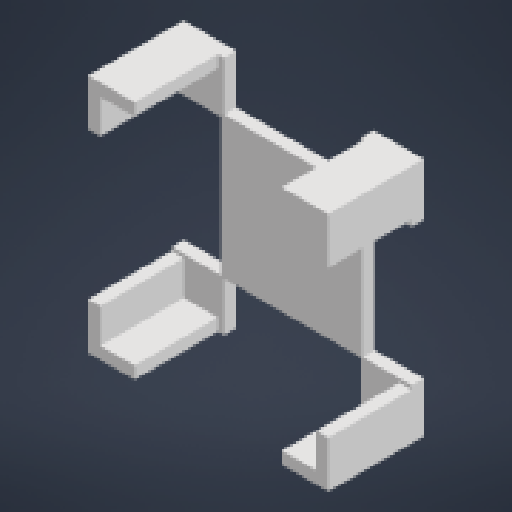
# Autodesk Inventor part: SistemaLiberacion2.2
Saved by Autodesk Inventor 2026.1 (Build 301233000, 233)
## iProperties
Created: 2025-11-13
Part Number: SistemaLiberacion2.2
Material: Genérico
Document SubType Name: Modeling
Designer: usuario
Density: 1 g/cm^3
Appearance: Valor por defecto
Author: usuario
Autodesk Inventor part; units mm, degrees
ref_plane "YZ Plane" through (0, 0, 0) normal (1, 0, 0) x (0, 1, 0)
ref_plane "XZ Plane" through (0, 0, 0) normal (0, 1, 0) x (-1, 0, 0)
ref_plane "XY Plane" through (0, 0, 0) normal (0, 0, 1) x (1, 0, 0)
sketch "Boceto1" plane through (0, 0, 0) normal (0, 0, 1) x (1, 0, 0)
  line L0 (-49, 49) -> (-49, -49)
  line L1 (-49, -49) -> (49, -49)
  line L2 (49, -49) -> (49, 49)
  line L3 (49, 49) -> (-49, 49)
  line L4 (-49, 49) -> (49, -49) construction
  line L5 (-49, -49) -> (49, 49) construction
  line L6 (-44, 44) -> (-44, -44)
  line L7 (-44, -44) -> (44, -44)
  line L8 (44, -44) -> (44, 44)
  line L9 (44, 44) -> (-44, 44)
  line L10 (-44, 44) -> (44, -44) construction
  line L11 (-44, -44) -> (44, 44) construction
  line L12 (-49, -30) -> (49, -30)
  line L13 (-49, 30) -> (49, 30)
  line L14 (-30, -49) -> (-30, 49)
  line L15 (30, -49) -> (30, 49)
  point P0 (0, 0)
  point P1 (0, -30)
  point P2 (0, -49)
  point P3 (-30, 44)
  point P4 (-44, 30)
  point P5 (30, 44)
  point P6 (44, 30)
  point P7 (30, -44)
  point P8 (44, -30)
  point P9 (-30, -44)
  point P10 (-44, -30)
  dimension "d0" = 98
  dimension "d1" = 98
  dimension "d2" = 5
  dimension "d3" = 5
  dimension "d8" = 19
  dimension "d10" = 19
  dimension "d11" = 19
  dimension "d18" = 19
  constraints: 32 end point, 8 point on line, 6 midpoint, 6 perpendicular, 4 parallel, 1 vertical
  measures "d0" distance of L0.start L0.end
  measures "d1" distance of L1.end L0.end
  measures "d2" distance between parallel lines of L1 L7
  measures "d3" distance between parallel lines of L8 L2
  measures "d8" distance of point (0, -30) point (0, -49)
  measures "d10" distance between parallel lines of L14 L0
  measures "d11" distance between parallel lines of L2 L15
  measures "d18" distance between parallel lines of L3 L13
extrude "Extrusión1" add sketch "Boceto1" against normal blind 34 contours L3 L14 L9 L6 L13 L0 | L12 L6 L7 L14 L1 L0 | L3 L2 L13 L8 L9 L15 | L15 L7 L8 L12 L2 L1
sketch "Boceto2" plane through (0, 0, -34) normal (0, 0, -1) x (-1, 0, 0)
  line L0 (49, 49) -> (-49, 49) projected
  line L1 (-49, -49) -> (49, -49) projected
  line L2 (-49, 49) -> (49, 49)
  line L3 (49, 49) -> (49, -49)
  line L4 (49, -49) -> (-49, -49)
  line L5 (-49, -49) -> (-49, 49)
  line L6 (49, -30) -> (44, -30) projected
  line L7 (49, 26) -> (49, -30)
  line L8 (-49, -30) -> (-49, 26)
  line L9 (30, 49) -> (-26, 49)
  line L10 (30, -49) -> (-30, -49)
  line L11 (-28.5, -49) -> (27.5, -49)
  line L12 (27.5, -49) -> (27.5, -34)
  line L13 (27.5, -34) -> (-28.5, -34)
  line L14 (-28.5, -34) -> (-28.5, -49)
  line L15 (-28.5, 34) -> (27.5, 34)
  line L16 (27.5, 34) -> (27.5, 49)
  line L17 (27.5, 49) -> (-28.5, 49)
  line L18 (-28.5, 49) -> (-28.5, 34)
  line L19 (-49, -28.5) -> (-34, -28.5)
  line L20 (-34, -28.5) -> (-34, 27.5)
  line L21 (-34, 27.5) -> (-49, 27.5)
  line L22 (-49, 27.5) -> (-49, -28.5)
  line L23 (34, -28.5) -> (49, -28.5)
  line L24 (49, -28.5) -> (49, 27.5)
  line L25 (49, 27.5) -> (34, 27.5)
  line L26 (34, 27.5) -> (34, -28.5)
  point P0 (0, 0)
  point P1 (-25.1585, 49)
  point P2 (24.6057, -49)
  point P3 (0, 49)
  point P4 (-0.5, 34)
  point P5 (-0.5, -34)
  dimension "d19" = 34
  dimension "d20" = 34
  dimension "d21" = 56
  dimension "d22" = 21.5
  dimension "d23" = 56
  dimension "d24" = 21.5
  dimension "d25" = 56
  dimension "d26" = 34
  dimension "d27" = 34
  constraints: 48 end point, 10 parallel, 7 horizontal, 6 point on line, 5 perpendicular, 4 collinear, 3 midpoint
  measures "d19" vertical distance of point (0, 0) point (-0.5, 34)
  measures "d20" vertical distance of point (-0.5, -34) point (0, 0)
  measures "d21" distance between parallel lines of L12 L14
  measures "d22" distance between parallel lines of L3 L12
  measures "d23" distance between parallel lines of L21 L19
  measures "d24" distance between parallel lines of L0 L21
  measures "d25" distance of L25.end L23.start
  measures "d26" distance from line of L26 point (0, 0)
  measures "d27" distance from line of point (0, 0) L20
extrude "Extrusión2" add sketch "Boceto2" along normal blind 5 contours L3 L25 L26 L23 L1 L12 L13 L14 L5 L19 L20 L21 L0 L18 L15 L16
